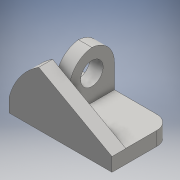
# Autodesk Inventor part: 240628_final2
Saved by Autodesk Inventor 2016 (Build 200138000, 138)
## iProperties
Created: 2024-06-28
Part Number: 240628_final2
Material: 일반
Document SubType Name: Modeling
Designer: pc
Density: 1 g/cm^3
Appearance: 기본값
Author: pc
Autodesk Inventor part; units mm, degrees
ref_plane "YZ Plane" through (0, 0, 0) normal (1, 0, 0) x (0, 1, 0)
ref_plane "XZ Plane" through (0, 0, 0) normal (0, 1, 0) x (-1, 0, 0)
ref_plane "XY Plane" through (0, 0, 0) normal (0, 0, 1) x (1, 0, 0)
sketch "스케치1" plane through (0, 0, 0) normal (0, 0, 1) x (1, 0, 0)
  line L0 (18.5261, -10.5982) -> (-18.5261, -10.5982)
  line L1 (-18.5261, -10.5982) -> (-18.5261, 10.5982)
  line L2 (-18.5261, 10.5982) -> (18.5261, 10.5982)
  line L3 (18.5261, 10.5982) -> (18.5261, -10.5982)
  line L4 (18.5261, -10.5982) -> (-18.5261, 10.5982) construction
  line L5 (-18.5261, -10.5982) -> (18.5261, 10.5982) construction
  point P0 (0, 0)
  constraints: 12 end point, 2 midpoint, 2 parallel, 1 horizontal, 1 perpendicular
extrude "돌출1" add sketch "스케치1" along normal blind 5
sketch "스케치2" plane through (0, 0, 5) normal (0, 0, 1) x (1, 0, 0)
  line L0 (-18.5261, -10.5982) -> (18.5261, -10.5982) projected
  line L1 (-18.5261, 10.5982) -> (-18.5261, -10.5982) projected
  line L2 (18.5261, -10.5982) -> (-18.5261, -10.5982)
  line L3 (-18.5261, -10.5982) -> (-18.5261, -5.5982)
  line L4 (-18.5261, -5.5982) -> (18.5261, -5.5982)
  line L5 (18.5261, -5.5982) -> (18.5261, -10.5982)
  point P0 (0, 0)
  dimension "d2" = 5
  constraints: 8 end point, 2 parallel, 1 horizontal, 1 perpendicular, 1 point on line
  measures "d2" distance of L2.end L3.end
extrude "돌출2" add sketch "스케치2" along normal blind 18.25
sketch "스케치3" plane through (-18.5261, -5.5982, 5) normal (0, 1, 0) x (1, 0, 0)
  line L0 (37.0522, 5) -> (37.0522, -18.25) projected
  line L1 (37.0522, 0.0749) -> (10.6495, -14.5756)
  line L2 (0, 5) -> (0, 0) projected
  arc A0 (0, 0) -> (10.6495, -14.5756) centre (23.9382, 6.3119) ccw
  line L3 (37.0522, 0.0749) -> (37.0522, -18.25)
  line L4 (37.0522, -18.25) -> (0, -18.25) projected
  line L5 (0, -18.25) -> (0, 0)
  point P0 (18.5261, 5)
  constraints: 6 end point, 2 point on circle, 1 centre point, 1 collinear, 1 perpendicular, 1 point on line
extrude "돌출3" cut sketch "스케치3" against normal blind 18.25
sketch "스케치4" plane through (0, 0, 5) normal (0, 0, 1) x (1, 0, 0)
  line L0 (-18.5261, -5.5982) -> (18.391, -5.5982) projected
  line L1 (18.5261, 10.5982) -> (-18.5261, 10.5982) projected
  line L2 (-1.8195, -5.5982) -> (-6.6451, -5.5982)
  line L3 (-6.6451, -5.5982) -> (-6.6451, 10.5982)
  line L4 (-6.6451, 10.5982) -> (-1.8195, 10.5982)
  line L5 (-1.8195, 10.5982) -> (-1.8195, -5.5982)
  point P0 (0, 0)
  constraints: 8 end point, 2 parallel, 2 point on line, 1 horizontal, 1 perpendicular
extrude "돌출4" add sketch "스케치4" along normal blind 17.25
sketch "스케치5" plane through (-6.6451, -5.5982, 5) normal (-1, 0, 0) x (0, 0, 1)
  arc A0 (9.1518, 0) -> (9.1518, 16.1965) centre (9.1518, 8.0982) ccw
  line L0 (0, 16.1965) -> (17.25, 16.1965) projected
  line L1 (17.25, 16.1965) -> (17.25, 0) projected
  circle A1 centre (9.1518, 8.0982) radius 4.0581
  line L2 (14.5756, 0) -> (0, 0) projected
  line L3 (0, 16.1965) -> (17.25, 16.1965) projected
  line L4 (9.1518, 16.1965) -> (17.25, 16.1965)
  line L5 (17.25, 16.1965) -> (17.25, 8.0982)
  line L6 (17.25, 0) -> (17.25, 16.1965) projected
  line L7 (17.25, 0) -> (9.1518, 0)
  line L8 (11.2145, 0) -> (17.25, 0) projected
  line L9 (17.25, 8.0982) -> (17.25, 0)
  line L10 (17.25, 0) -> (9.1518, 0)
  point P0 (-5, 5.5982)
  constraints: 10 end point, 6 tangent, 3 collinear, 2 centre point, 2 point on circle, 2 point on line, 1 coincident, 1 midpoint, 1 vertical
extrude "돌출5" cut sketch "스케치5" against normal blind 17.25 contours A1
sketch "스케치6" plane through (-1.8195, -5.5982, 5) normal (1, 0, 0) x (0, 0, -1)
  line L0 (-17.25, 16.1965) -> (-17.25, 0) projected
  line L1 (0, 16.1965) -> (-17.25, 16.1965) projected
  line L2 (-17.25, 8.0982) -> (-17.25, 16.1965)
  line L3 (-17.25, 16.1965) -> (-8.625, 16.1965)
  line L4 (-17.25, 0) -> (-17.25, 8.0982)
  line L5 (-11.2145, 0) -> (-17.25, 0) projected
  line L6 (-17.25, 0) -> (-8.3415, 0)
  line L7 (0, 0) -> (-14.5756, 0) projected
  arc A0 (-17.25, 8.0982) -> (-8.3415, 0) centre (-8.3415, 8.949) ccw
  arc A1 (-8.625, 16.1965) -> (-17.25, 8.0982) centre (-8.625, 7.5543) ccw
  point P0 (5, 5.5982)
  constraints: 8 end point, 4 point on circle, 2 centre point, 2 midpoint, 2 tangent, 1 collinear, 1 point on line, 1 vertical
extrude "돌출6" cut sketch "스케치6" against normal blind 17.25
fillet "모깎기1" radius 5 2 edges at (-18.5261, 10.5982, 2.5) (18.5261, 10.5982, 2.5)
